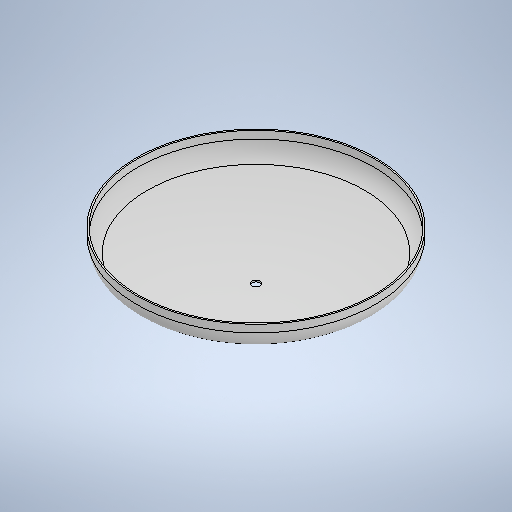
# Autodesk Inventor part: Сферическое дно D1000
Saved by Autodesk Inventor 2025.1 (Build 291241020, 241B)
## iProperties
Created: 2025-02-16
Part Number: Сферическое дно D1000
Material: Generic
Document SubType Name: Modeling
Designer: pokla
Density: 1 g/cm^3
Appearance: Default
Author: pokla
Autodesk Inventor part; units mm, degrees
ref_plane "YZ Plane" through (0, 0, 0) normal (1, 0, 0) x (0, 1, 0)
ref_plane "XZ Plane" through (0, 0, 0) normal (0, 1, 0) x (-1, 0, 0)
ref_plane "XY Plane" through (0, 0, 0) normal (0, 0, 1) x (1, 0, 0)
sketch "Sketch1" plane through (0, 0, 0) normal (0, 1, 0) x (-1, 0, 0)
  line L0 (477.5, 0) -> (477.5, -30)
  arc A0 (437, -96.5939) -> (477.5, -30) centre (402.5, -30) ccw
  arc A1 (0, -203.0709) -> (437, -96.5939) centre (0, 746.9291) ccw
  line L1 (0, 191.6842) -> (0, -191.6842)
  arc A2 (0, -197.0709) -> (434.24, -91.2664) centre (0, 746.9291) ccw
  arc A3 (434.24, -91.2664) -> (471.5, -30) centre (402.5, -30) ccw
  line L2 (471.5, -30) -> (471.5, 0)
  line L3 (471.5, 0) -> (477.5, 0)
  line L4 (0, -197.0709) -> (0, -203.0709)
  point P0 (0, 0)
  point P1 (0, 0)
  point P2 (0, -200.0709)
  point P3 (0, -158.7016)
  point P4 (0, -164.7016)
  dimension "d0" = 75
  dimension "d1" = 30
  dimension "d3" = 950
  dimension "d6" = 6
  dimension "d12" = 943
  constraints: 10 end point, 8 point on circle, 4 centre point, 2 midpoint, 2 tangent, 2 vertical, 1 coincident, 1 horizontal, 1 horizontal alignment, 1 line through centre, 1 parallel, 1 vertical alignment, 2 other
  measures "d0" radius of A0
  measures "d1" distance of L0.start L0.end
  measures "d3" radius of A1
  measures "d6" radial gap between concentric circles of A1 A2
  measures "d12" diameter of L2 L1
revolve "Revolution1" add sketch "Sketch1" angle 360 about axis through (0, 0, 191.6842) along (0, 0, -1)
sketch "Sketch2" plane through (0, 0, 0) normal (0, 0, 1) x (1, 0, 0)
  circle A0 centre (0, 0) radius 16.75
  dimension "d8" = 33.5
  constraints: 1 centre point, 1 coincident
  measures "d8" diameter of A0
extrude "Extrusion1" cut sketch "Sketch2" against normal through all
body "Solid1"
